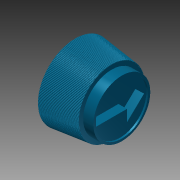
# Autodesk Inventor part: PerillaPotenciometro
Saved by Autodesk Inventor 2013 (Build 170138000, 138)
## iProperties
Created: 2013-06-26
Part Number: PerillaPotenciometro
Material: Genérico
Document SubType Name: Modeling
Designer: usuario
Density: 1 g/cm^3
Author: usuario
Autodesk Inventor part; units mm, degrees
ref_plane "XZ Plane" through (0, 0, 0) normal (0, 1, 0) x (-1, 0, 0)
ref_plane "XY Plane" through (0, 0, 0) normal (0, 0, 1) x (1, 0, 0)
sketch "Boceto4" plane through (0, 0, 0) normal (1, 0, 0) x (0, 1, 0)
  circle A0 centre (0, 0) radius 4.3
  dimension "d4" = 8.6
  constraints: 1 centre point, 1 coincident
  measures "d4" diameter of A0
ref_plane "Plano de trabajo1" through (4.26, 0, 0) normal (1, 0, 0) x (0, 1, 0)
sketch "Boceto5" plane through (4.26, 0, 0) normal (1, 0, 0) x (0, 1, 0)
  circle A0 centre (0, 0) radius 3.8
  dimension "d6" = 7.6
  constraints: 1 centre point, 1 coincident
  measures "d6" diameter of A0
loft "Solevación1" add profiles "Boceto4", "Boceto5"
sketch "Boceto6" plane through (4.26, 0, 0) normal (1, 0, 0) x (0, 0, -1)
  circle A0 centre (0, 0) radius 3.8 projected
  circle A1 centre (0, 0) radius 3.32
  dimension "d11" = 6.64
  constraints: 1 centre point, 1 coincident
  measures "d11" diameter of A1
extrude "Extrusión2" add sketch "Boceto6" along normal blind 1.2 contours A1
hole "Hole1" at (5.46, 0, 0) direction (-1, 0, 0) diameter 6.12 depth 0.2
sketch "Boceto7" plane through (0, 0, 0) normal (-1, 0, 0) x (0, 0, 1)
  circle A0 centre (0, 0) radius 4.3 projected
  circle A1 centre (0, 0) radius 0.5
  dimension "d23" = 1
  constraints: 1 centre point, 1 coincident
  measures "d23" diameter of A1
extrude "Extrusión3" add sketch "Boceto7" along normal blind 1.98 contours A1
sketch "Boceto8" plane through (5.26, 0, 0) normal (1, 0, 0) x (0, 0, -1)
  circle A0 centre (0, 0) radius 3.06 projected
  line L0 (0.55, 2.8) -> (-0.55, 2.8)
  line L1 (-0.55, 2.8) -> (-0.55, -2.8)
  line L2 (-0.55, -2.8) -> (0.55, -2.8)
  line L3 (0.55, -2.8) -> (0.55, 2.8)
  line L4 (0.55, 2.8) -> (-0.55, -2.8) construction
  line L5 (-0.55, 2.8) -> (0.55, -2.8) construction
  dimension "d26" = 1.1
  dimension "d27" = 5.6
  constraints: 12 end point, 2 midpoint, 2 parallel, 1 horizontal, 1 perpendicular
  measures "d26" distance of L2.end L1.end
  measures "d27" distance of L1.end L0.end
extrude "Extrusión4" cut sketch "Boceto8" against normal blind 1 contours L3 L2 L1 L0
sketch "Boceto9" plane through (5.26, 0, 0) normal (1, 0, 0) x (0, 0, -1)
  line L0 (-0.55, 2.8) -> (0.55, 2.8) projected
  line L1 (0, 0.8) -> (1.9, 0.8)
  line L2 (1.9, 0.8) -> (0, 2.8)
  line L3 (0, 0.8) -> (-1.9, 0.8)
  line L4 (-1.9, 0.8) -> (0, 2.8)
  dimension "d30" = 2
  dimension "d31" = 1.9
  dimension "d32" = 1.9
  constraints: 8 end point, 1 collinear, 1 midpoint
  measures "d30" distance of L2.end L1.start
  measures "d31" distance of L1.start L1.end
  measures "d32" distance of L1.start L3.end
extrude "Extrusión5" cut sketch "Boceto9" against normal blind 1
sketch "Boceto10" plane through (5.26, 0, 0) normal (1, 0, 0) x (0, 0, -1)
  line L0 (0.55, 2.2211) -> (1.9, 0.8) projected
  line L1 (-0.55, 2.2211) -> (-0.55, 2.8) projected
  line L2 (-0.55, 2.8) -> (0.55, 2.8) projected
  line L3 (0.55, 2.8) -> (0.55, 2.2211) projected
  line L4 (-0.55, 2.2211) -> (0, 2.8)
  line L5 (0, 2.8) -> (0.55, 2.2211)
  line L6 (0.55, 2.2211) -> (0.55, 2.8)
  line L7 (0.55, 2.8) -> (0, 2.8)
  line L8 (-0.55, 2.8) -> (-0.55, 2.2211)
  line L9 (-0.55, 2.8) -> (0, 2.8)
  constraints: 12 end point, 5 collinear, 1 midpoint
extrude "Extrusión6" add sketch "Boceto10" against normal blind 1
sketch "Boceto11" plane through (4.26, 0, 0) normal (1, 0, 0) x (0, 0, -1)
  circle A0 centre (3.8, 0) radius 0.05
  dimension "d37" = 0.1
  constraints: 1 centre point
  measures "d37" diameter of A0
sketch "Boceto12" plane through (0, 0, 0) normal (-1, 0, 0) x (0, 0, 1)
  circle A0 centre (-4.3, 0) radius 0.05
  dimension "d38" = 0.1
  constraints: 1 centre point
  measures "d38" diameter of A0
loft "Solevación2" add profiles "Boceto11", "Boceto12"
pattern_circular "Patrón circular1" count 200 over 360 about axis through (0, 0, 0) along (1, 0, 0) of "Solevación2"
